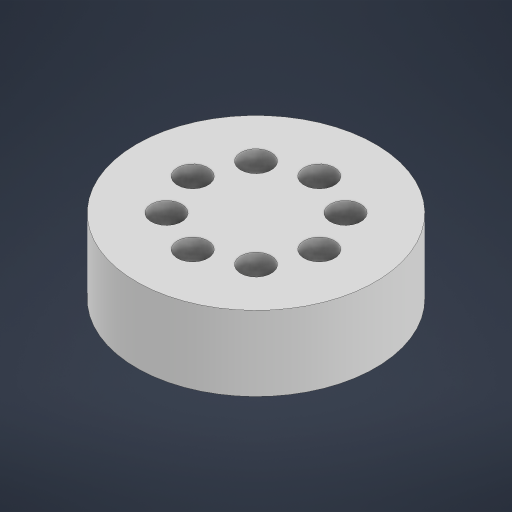
# Autodesk Inventor part: PulleySpacer
Saved by Autodesk Inventor 2024 (Build 280153000, 153)
## iProperties
Created: 2023-10-18
Part Number: PulleySpacer
Material: Generic
Document SubType Name: Modeling
Designer: avsar
Density: 1 g/cm^3
Appearance: Default
Author: avsar
Autodesk Inventor part; units mm, degrees
ref_plane "YZ Plane" through (0, 0, 0) normal (1, 0, 0) x (0, 1, 0)
ref_plane "XZ Plane" through (0, 0, 0) normal (0, 1, 0) x (-1, 0, 0)
ref_plane "XY Plane" through (0, 0, 0) normal (0, 0, 1) x (1, 0, 0)
sketch "Sketch1" plane through (0, 0, 0) normal (0, 1, 0) x (-1, 0, 0)
  circle A0 centre (0, 0) radius 16
  circle A1 centre (0, 0) radius 2.5 construction
  circle A2 centre (6, 6) radius 2.05
  circle A3 centre (0, 8.4853) radius 2.05
  circle A4 centre (-6, 6) radius 2.05
  circle A5 centre (-8.4853, 0) radius 2.05
  circle A6 centre (-6, -6) radius 2.05
  circle A7 centre (0, -8.4853) radius 2.05
  circle A8 centre (6, -6) radius 2.05
  circle A9 centre (8.4853, 0) radius 2.05
  dimension "d0" = 32
  dimension "d1" = 5
  dimension "d2" = 4.1
  dimension "d3" = 6
  dimension "d4" = 6
  dimension "d7" = 360
  constraints: 10 centre point, 2 coincident, 17 other
  measures "d0" diameter of A0
  measures "d1" diameter of A1
  measures "d2" diameter of A2
  measures "d3" horizontal distance of point (0, 0) A2.centre
  measures "d4" horizontal distance of point (0, 0) A2.centre
extrude "Extrusion1" add sketch "Sketch1" along normal mid plane 10
body "Solid1"
